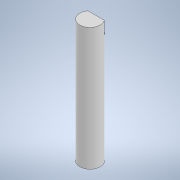
# Autodesk Inventor part: Ось колес
Saved by Autodesk Inventor 2020 (Build 240168000, 168)
## iProperties
Created: 2021-02-28
Part Number: Ось колес
Material: Типовые
Document SubType Name: Modeling
Designer: Антон
Density: 1 g/cm^3
Appearance: По умолчанию
Author: Антон
Autodesk Inventor part; units mm, degrees
ref_plane "YZ Plane" through (0, 0, 0) normal (1, 0, 0) x (0, 1, 0)
ref_plane "XZ Plane" through (0, 0, 0) normal (0, 1, 0) x (-1, 0, 0)
ref_plane "XY Plane" through (0, 0, 0) normal (0, 0, 1) x (1, 0, 0)
sketch "Эскиз1" plane through (0, 0, 0) normal (0, 1, 0) x (-1, 0, 0)
  circle A0 centre (0, 0) radius 2.5
  dimension "d0" = 5
  constraints: 1 centre point, 1 coincident
  measures "d0" diameter of A0
extrude "Выдавливание1" add sketch "Эскиз1" along normal mid plane 30
sketch "Эскиз2" plane through (0, 15, 0) normal (0, 1, 0) x (1, 0, 0)
  circle A0 centre (0, 0) radius 2.5
  line L0 (2.5, -1.5) -> (-2.5, -1.5)
  line L1 (-2.5, -1.5) -> (-2.5, 1.5)
  line L2 (-2.5, 1.5) -> (2.5, 1.5)
  line L3 (2.5, 1.5) -> (2.5, -1.5)
  line L4 (2.5, -1.5) -> (-2.5, 1.5) construction
  line L5 (-2.5, -1.5) -> (2.5, 1.5) construction
  point P0 (-2, 1.5)
  point P1 (2, 1.5)
  dimension "d3" = 5
  dimension "d4" = 3
  constraints: 12 end point, 2 midpoint, 2 parallel, 1 centre point, 1 coincident, 1 horizontal, 1 perpendicular
  measures "d3" distance of L1.end L2.end
  measures "d4" distance of L0.end L1.end
extrude "Выдавливание2" cut sketch "Эскиз2" against normal blind 3 contours L2 A0
